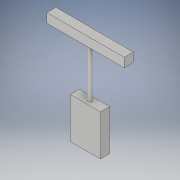
# Autodesk Inventor part: switchbox
Saved by Autodesk Inventor 2019 (Build 230136000, 136)
## iProperties
Created: 2018-07-11
Part Number: switchbox
Material: Generic
Document SubType Name: Modeling
Designer: User
Density: 1 g/cm^3
Appearance: Aluminum - Polished
Author: User
Autodesk Inventor part; units mm, degrees
ref_plane "YZ Plane" through (0, 0, 0) normal (1, 0, 0) x (0, 1, 0)
ref_plane "XZ Plane" through (0, 0, 0) normal (0, 1, 0) x (-1, 0, 0)
ref_plane "XY Plane" through (0, 0, 0) normal (0, 0, 1) x (1, 0, 0)
sketch "Sketch1" plane through (0, 0, 0) normal (0, 0, 1) x (1, 0, 0)
  line L0 (-177.8, -241.3) -> (177.8, -241.3)
  line L1 (177.8, -241.3) -> (177.8, 241.3)
  line L2 (177.8, 241.3) -> (-177.8, 241.3)
  line L3 (-177.8, 241.3) -> (-177.8, -241.3)
  line L4 (-177.8, -241.3) -> (177.8, 241.3) construction
  line L5 (177.8, -241.3) -> (-177.8, 241.3) construction
  point P0 (0, 0)
  dimension "d0" = 355.6
  dimension "d1" = 482.6
  constraints: 12 end point, 2 midpoint, 2 parallel, 1 horizontal, 1 perpendicular
  measures "d0" distance of L1.end L2.end
  measures "d1" distance of L0.end L1.end
extrude "Extrusion1" add sketch "Sketch1" along normal blind 107.95
sketch "Sketch2" plane through (-177.8, 241.3, 0) normal (0, 1, 0) x (1, 0, 0)
  line L0 (355.6, 0) -> (0, 0) projected
  line L1 (0, 0) -> (0, -107.95) projected
  line L2 (355.6, -107.95) -> (0, -107.95) projected
  line L3 (355.6, 0) -> (355.6, -107.95) projected
  circle A0 centre (177.8, -53.975) radius 22.225
  line L4 (177.8, -53.975) -> (177.8, -107.95) construction
  line L5 (0, -107.95) -> (355.6, -107.95) projected
  line L6 (177.8, -53.975) -> (355.6, -53.975) construction
  point P0 (177.8, 0)
  dimension "d4" = 44.45
  constraints: 4 end point, 2 midpoint, 2 perpendicular, 1 centre point
  measures "d4" diameter of A0
extrude "Extrusion2" add sketch "Sketch2" along normal blind 590.55 contours A0
sketch "Sketch3" plane through (0, 831.85, 53.975) normal (0, 1, 0) x (1, 0, 0)
  circle A0 centre (0, 0) radius 22.225 projected
  line L0 (-457.2, 53.975) -> (457.2, 53.975)
  line L1 (457.2, 53.975) -> (457.2, -53.975)
  line L2 (457.2, -53.975) -> (-457.2, -53.975)
  line L3 (-457.2, -53.975) -> (-457.2, 53.975)
  circle A1 centre (0, 0) radius 22.225 projected
  line L4 (177.8, 53.975) -> (-177.8, 53.975) projected
  line L5 (-177.8, 53.975) -> (-177.8, -53.975) projected
  line L6 (177.8, -53.975) -> (-177.8, -53.975) projected
  line L7 (177.8, 53.975) -> (177.8, -53.975) projected
  line L8 (0, 0) -> (0, 53.975) construction
  point P0 (0, 53.975)
  dimension "d7" = 914.4
  dimension "d10" = 107.95
  constraints: 10 end point, 2 parallel, 2 perpendicular, 1 collinear, 1 horizontal, 1 midpoint
  measures "d7" distance of L0.start L0.end
  measures "d10" distance of L2.end L0.start
extrude "Extrusion3" add sketch "Sketch3" along normal blind 107.95 contours A0 | L0 L5 L2 L3 | L0 L7 L2 L5 | L0 L1 L2 L7
body "Solid1"
